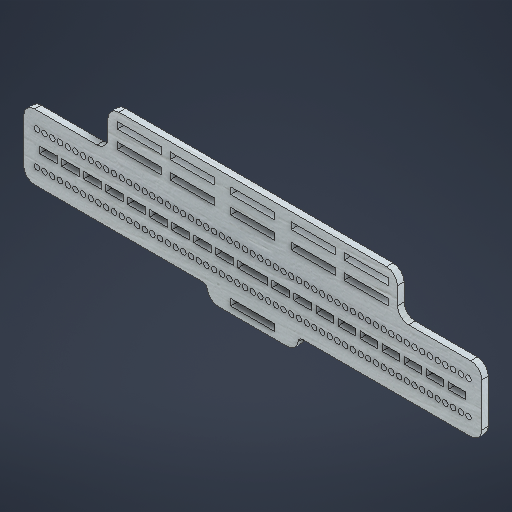
# Autodesk Inventor part: side_frame_test
Saved by Autodesk Inventor 2025.3 (Build 293356030, 356C)
## iProperties
Created: 2025-09-04
Part Number: side_frame_test
Material: 木材 (楓木)
Document SubType Name: Modeling
Designer: 陳泓任
Density: 0.67 g/cm^3
Appearance: 木材 - 白色刷漆
Author: 陳泓任
Autodesk Inventor part; units mm, degrees
ref_plane "YZ Plane" through (0, 0, 0) normal (1, 0, 0) x (0, 1, 0)
ref_plane "XZ Plane" through (0, 0, 0) normal (0, 1, 0) x (-1, 0, 0)
ref_plane "XY Plane" through (0, 0, 0) normal (0, 0, 1) x (1, 0, 0)
sketch "草圖1" plane through (0, 0, 0) normal (0, 0, 1) x (1, 0, 0)
  line L0 (41.49, 17.7685) -> (41.49, 20.7685)
  line L1 (41.49, 20.7685) -> (61.49, 20.7685)
  line L2 (61.49, 20.7685) -> (61.49, 17.7685)
  line L3 (61.49, 17.7685) -> (41.49, 17.7685)
  arc A0 (99, -14.8985) -> (104, -9.8985) centre (99, -9.8985) ccw
  arc A1 (-104, -9.8985) -> (-99, -14.8985) centre (-99, -9.8985) ccw
  line L4 (-61.49, 17.7685) -> (-61.49, 20.7685)
  line L5 (-61.49, 20.7685) -> (-41.49, 20.7685)
  line L6 (-41.49, 20.7685) -> (-41.49, 17.7685)
  line L7 (-41.49, 17.7685) -> (-61.49, 17.7685)
  arc A2 (65.74, 27.7685) -> (60.74, 32.7685) centre (60.74, 27.7685) ccw
  circle A3 centre (0, 7.5) radius 1.25
  circle A4 centre (0, -7.5) radius 1.25
  arc A5 (-70.74, 14.8985) -> (-65.74, 19.8985) centre (-70.74, 19.8985) ccw
  arc A6 (104, 9.8985) -> (99, 14.8985) centre (99, 9.8985) ccw
  arc A7 (-99, 14.8985) -> (-104, 9.8985) centre (-99, 9.8985) ccw
  arc A8 (65.74, 19.8985) -> (70.74, 14.8985) centre (70.74, 19.8985) ccw
  line L8 (-99, -14.8985) -> (-22.615, -14.8985)
  arc A9 (15.6624, -21.0852) -> (20.6286, -16.6661) centre (15.6624, -16.0852) ccw
  arc A10 (22.615, -14.8985) -> (20.6286, -16.6661) centre (22.615, -16.8985) ccw
  line L9 (-10, -18.0852) -> (-10, -15.0852)
  line L10 (-10, -15.0852) -> (10, -15.0852)
  line L11 (10, -15.0852) -> (10, -18.0852)
  line L12 (10, -18.0852) -> (-10, -18.0852)
  arc A11 (-20.6286, -16.6661) -> (-22.615, -14.8985) centre (-22.615, -16.8985) ccw
  arc A12 (-20.6286, -16.6661) -> (-15.6624, -21.0852) centre (-15.6624, -16.0852) ccw
  line L13 (-65.74, 27.7685) -> (-65.74, 19.8985)
  line L14 (-104, 9.8985) -> (-104, -9.8985)
  line L15 (104, 9.8985) -> (104, -9.8985)
  line L16 (-15.6624, -21.0852) -> (15.6624, -21.0852)
  line L17 (22.615, -14.8985) -> (99, -14.8985)
  line L18 (70.74, 14.8985) -> (99, 14.8985)
  line L19 (-99, 14.8985) -> (-70.74, 14.8985)
  line L20 (0, -35.3826) -> (0, 51.5191) construction
  line L21 (-104.9871, 0) -> (119.3176, 0) construction
  line L22 (65.74, 27.7685) -> (65.74, 19.8985)
  line L23 (0, 7.5) -> (0, -7.5)
  line L24 (-60.74, 32.7685) -> (60.74, 32.7685)
  arc A13 (-60.74, 32.7685) -> (-65.74, 27.7685) centre (-60.74, 27.7685) ccw
  line L25 (-61.49, 28.7685) -> (-41.49, 28.7685)
  line L26 (-61.49, 25.7685) -> (-61.49, 28.7685)
  line L27 (-41.49, 25.7685) -> (-61.49, 25.7685)
  line L28 (-41.49, 28.7685) -> (-41.49, 25.7685)
  line L29 (41.49, 28.7685) -> (61.49, 28.7685)
  line L30 (41.49, 25.7685) -> (41.49, 28.7685)
  line L31 (61.49, 25.7685) -> (41.49, 25.7685)
  line L32 (61.49, 28.7685) -> (61.49, 25.7685)
  line L33 (-17.49, 28.7685) -> (-17.49, 25.7685)
  line L34 (-17.49, 25.7685) -> (-37.49, 25.7685)
  line L35 (-37.49, 28.7685) -> (-17.49, 28.7685)
  line L36 (-37.49, 25.7685) -> (-37.49, 28.7685)
  line L37 (-17.49, 20.7685) -> (-17.49, 17.7685)
  line L38 (-17.49, 17.7685) -> (-37.49, 17.7685)
  line L39 (-37.49, 20.7685) -> (-17.49, 20.7685)
  line L40 (-37.49, 17.7685) -> (-37.49, 20.7685)
  line L41 (17.49, 28.7685) -> (17.49, 25.7685)
  line L42 (17.49, 25.7685) -> (37.49, 25.7685)
  line L43 (37.49, 28.7685) -> (17.49, 28.7685)
  line L44 (37.49, 25.7685) -> (37.49, 28.7685)
  line L45 (17.49, 20.7685) -> (17.49, 17.7685)
  line L46 (17.49, 17.7685) -> (37.49, 17.7685)
  line L47 (37.49, 20.7685) -> (17.49, 20.7685)
  line L48 (37.49, 17.7685) -> (37.49, 20.7685)
  line L49 (10, 28.7685) -> (10, 25.7685)
  line L50 (10, 25.7685) -> (-10, 25.7685)
  line L51 (-10, 28.7685) -> (10, 28.7685)
  line L52 (-10, 25.7685) -> (-10, 28.7685)
  line L53 (10, 20.7685) -> (10, 17.7685)
  line L54 (10, 17.7685) -> (-10, 17.7685)
  line L55 (-10, 20.7685) -> (10, 20.7685)
  line L56 (-10, 17.7685) -> (-10, 20.7685)
  circle A14 centre (3.5, 7.5) radius 1.25
  circle A15 centre (3.5, -7.5) radius 1.25
  circle A16 centre (-3.5, 7.5) radius 1.25
  circle A17 centre (-3.5, -7.5) radius 1.25
  circle A18 centre (7, 7.5) radius 1.25
  circle A19 centre (7, -7.5) radius 1.25
  circle A20 centre (-7, 7.5) radius 1.25
  circle A21 centre (-7, -7.5) radius 1.25
  circle A22 centre (10.5, 7.5) radius 1.25
  circle A23 centre (10.5, -7.5) radius 1.25
  circle A24 centre (-10.5, 7.5) radius 1.25
  circle A25 centre (-10.5, -7.5) radius 1.25
  circle A26 centre (14, 7.5) radius 1.25
  circle A27 centre (14, -7.5) radius 1.25
  circle A28 centre (-14, 7.5) radius 1.25
  circle A29 centre (-14, -7.5) radius 1.25
  circle A30 centre (17.5, 7.5) radius 1.25
  circle A31 centre (17.5, -7.5) radius 1.25
  circle A32 centre (-17.5, 7.5) radius 1.25
  circle A33 centre (-17.5, -7.5) radius 1.25
  circle A34 centre (21, 7.5) radius 1.25
  circle A35 centre (21, -7.5) radius 1.25
  circle A36 centre (-21, 7.5) radius 1.25
  circle A37 centre (-21, -7.5) radius 1.25
  circle A38 centre (24.5, 7.5) radius 1.25
  circle A39 centre (24.5, -7.5) radius 1.25
  circle A40 centre (-24.5, 7.5) radius 1.25
  circle A41 centre (-24.5, -7.5) radius 1.25
  circle A42 centre (28, 7.5) radius 1.25
  circle A43 centre (28, -7.5) radius 1.25
  circle A44 centre (-28, 7.5) radius 1.25
  circle A45 centre (-28, -7.5) radius 1.25
  circle A46 centre (31.5, 7.5) radius 1.25
  circle A47 centre (31.5, -7.5) radius 1.25
  circle A48 centre (-31.5, 7.5) radius 1.25
  circle A49 centre (-31.5, -7.5) radius 1.25
  circle A50 centre (35, 7.5) radius 1.25
  circle A51 centre (35, -7.5) radius 1.25
  circle A52 centre (-35, 7.5) radius 1.25
  circle A53 centre (-35, -7.5) radius 1.25
  circle A54 centre (38.5, 7.5) radius 1.25
  circle A55 centre (38.5, -7.5) radius 1.25
  circle A56 centre (-38.5, 7.5) radius 1.25
  circle A57 centre (-38.5, -7.5) radius 1.25
  circle A58 centre (42, 7.5) radius 1.25
  circle A59 centre (42, -7.5) radius 1.25
  circle A60 centre (-42, 7.5) radius 1.25
  circle A61 centre (-42, -7.5) radius 1.25
  circle A62 centre (45.5, 7.5) radius 1.25
  circle A63 centre (45.5, -7.5) radius 1.25
  circle A64 centre (-45.5, 7.5) radius 1.25
  circle A65 centre (-45.5, -7.5) radius 1.25
  circle A66 centre (49, 7.5) radius 1.25
  circle A67 centre (49, -7.5) radius 1.25
  circle A68 centre (-49, 7.5) radius 1.25
  circle A69 centre (-49, -7.5) radius 1.25
  circle A70 centre (52.5, 7.5) radius 1.25
  circle A71 centre (52.5, -7.5) radius 1.25
  circle A72 centre (-52.5, 7.5) radius 1.25
  circle A73 centre (-52.5, -7.5) radius 1.25
  circle A74 centre (56, 7.5) radius 1.25
  circle A75 centre (56, -7.5) radius 1.25
  circle A76 centre (-56, 7.5) radius 1.25
  circle A77 centre (-56, -7.5) radius 1.25
  circle A78 centre (59.5, 7.5) radius 1.25
  circle A79 centre (59.5, -7.5) radius 1.25
  circle A80 centre (-59.5, 7.5) radius 1.25
  circle A81 centre (-59.5, -7.5) radius 1.25
  circle A82 centre (63, 7.5) radius 1.25
  circle A83 centre (63, -7.5) radius 1.25
  circle A84 centre (-63, 7.5) radius 1.25
  circle A85 centre (-63, -7.5) radius 1.25
  circle A86 centre (66.5, 7.5) radius 1.25
  circle A87 centre (66.5, -7.5) radius 1.25
  circle A88 centre (-66.5, 7.5) radius 1.25
  circle A89 centre (-66.5, -7.5) radius 1.25
  circle A90 centre (70, 7.5) radius 1.25
  circle A91 centre (70, -7.5) radius 1.25
  circle A92 centre (-70, 7.5) radius 1.25
  circle A93 centre (-70, -7.5) radius 1.25
  circle A94 centre (73.5, 7.5) radius 1.25
  circle A95 centre (73.5, -7.5) radius 1.25
  circle A96 centre (-73.5, 7.5) radius 1.25
  circle A97 centre (-73.5, -7.5) radius 1.25
  circle A98 centre (77, 7.5) radius 1.25
  circle A99 centre (77, -7.5) radius 1.25
  circle A100 centre (-77, 7.5) radius 1.25
  circle A101 centre (-77, -7.5) radius 1.25
  circle A102 centre (80.5, 7.5) radius 1.25
  circle A103 centre (80.5, -7.5) radius 1.25
  circle A104 centre (-80.5, 7.5) radius 1.25
  circle A105 centre (-80.5, -7.5) radius 1.25
  circle A106 centre (84, 7.5) radius 1.25
  circle A107 centre (84, -7.5) radius 1.25
  circle A108 centre (-84, 7.5) radius 1.25
  circle A109 centre (-84, -7.5) radius 1.25
  circle A110 centre (87.5, 7.5) radius 1.25
  circle A111 centre (87.5, -7.5) radius 1.25
  circle A112 centre (-87.5, 7.5) radius 1.25
  circle A113 centre (-87.5, -7.5) radius 1.25
  circle A114 centre (91, 7.5) radius 1.25
  circle A115 centre (91, -7.5) radius 1.25
  circle A116 centre (-91, 7.5) radius 1.25
  circle A117 centre (-91, -7.5) radius 1.25
  circle A118 centre (94.5, 7.5) radius 1.25
  circle A119 centre (94.5, -7.5) radius 1.25
  circle A120 centre (-94.5, 7.5) radius 1.25
  circle A121 centre (-94.5, -7.5) radius 1.25
  circle A122 centre (98, 7.5) radius 1.25
  circle A123 centre (98, -7.5) radius 1.25
  circle A124 centre (-98, 7.5) radius 1.25
  circle A125 centre (-98, -7.5) radius 1.25
  point P0 (0, 0)
  point P1 (-65.74, 32.7685)
  point P2 (0, -15.0852)
  point P3 (-104, 0)
  point P4 (0, 32.7638)
  point P5 (-36.74, 27.7685)
  dimension "d0" = 20
  dimension "d1" = 3
  dimension "d2" = 3
  dimension "d4" = 2.5
  dimension "d7" = 4.25
  dimension "d11" = 5
  dimension "d12" = 2
  dimension "d16" = 15
  dimension "d26" = 29.797
  dimension "d29" = 45.23
  dimension "d30" = 31.3249
  dimension "d43" = 208
  dimension "d44" = 4.25
  dimension "d45" = 5
  dimension "d46" = 17.87
  dimension "d48" = 38.26
  dimension "d49" = 12
  dimension "d54" = 8
  dimension "d61" = 24
  dimension "d92" = 3.5
  constraints: 126 centre point, 114 end point, 24 point on circle, 22 tangent, 11 collinear, 10 equal length, 10 equal radius, 8 symmetric about line, 7 horizontal, 7 point on line, 5 perpendicular, 5 vertical, 2 midpoint, 262 other
  measures "d0" distance of L11.end L9.start
  measures "d1" distance of L9.start L9.end
  measures "d2" distance between parallel lines of L16 L12
  measures "d4" diameter of A3
  measures "d7" distance between parallel lines of L13 L4
  measures "d11" radius of A2
  measures "d12" radius of A11
  measures "d16" distance of L23.end L23.start
  measures "d26" distance between parallel lines of L18 L17
  measures "d29" distance of A10.centre A11.centre
  measures "d30" distance of L16.start L16.end
  measures "d43" diameter of L14 L20
  measures "d44" distance between parallel lines of L22 L2
  measures "d45" radius of A13
  measures "d46" distance between parallel lines of L19 L24
  measures "d48" distance between parallel lines of L22 L15
  measures "d49" distance between parallel lines of L5 L24
  measures "d54" distance of L4.end L25.start
  measures "d61" distance of L27.start L33.end
  measures "d92" distance of L23.start A14.centre
extrude "擠出1" add sketch "草圖1" along normal blind 3
sketch "草圖2" plane through (0, 0, 3) normal (0, 0, 1) x (1, 0, 0)
  line L0 (-104.9871, 0) -> (119.3176, 0) projected
  line L1 (0, -35.3826) -> (0, 51.5191) projected
  line L2 (-1.25, 1.5) -> (6.75, 1.5)
  line L3 (6.75, 1.5) -> (6.75, -1.5)
  line L4 (6.75, -1.5) -> (-1.25, -1.5)
  line L5 (-1.25, -1.5) -> (-1.25, 1.5)
  circle A0 centre (0, 7.5) radius 1.25 projected
  circle A1 centre (0, -7.5) radius 1.25 projected
  line L6 (8.75, 1.5) -> (16.75, 1.5)
  line L7 (16.75, -1.5) -> (8.75, -1.5)
  line L8 (8.75, -1.5) -> (8.75, 1.5)
  line L9 (16.75, 1.5) -> (16.75, -1.5)
  line L10 (18.75, 1.5) -> (26.75, 1.5)
  line L11 (26.75, -1.5) -> (18.75, -1.5)
  line L12 (18.75, -1.5) -> (18.75, 1.5)
  line L13 (26.75, 1.5) -> (26.75, -1.5)
  line L14 (28.75, 1.5) -> (36.75, 1.5)
  line L15 (36.75, -1.5) -> (28.75, -1.5)
  line L16 (28.75, -1.5) -> (28.75, 1.5)
  line L17 (36.75, 1.5) -> (36.75, -1.5)
  line L18 (38.75, 1.5) -> (46.75, 1.5)
  line L19 (46.75, -1.5) -> (38.75, -1.5)
  line L20 (38.75, -1.5) -> (38.75, 1.5)
  line L21 (46.75, 1.5) -> (46.75, -1.5)
  line L22 (48.75, 1.5) -> (56.75, 1.5)
  line L23 (56.75, -1.5) -> (48.75, -1.5)
  line L24 (48.75, -1.5) -> (48.75, 1.5)
  line L25 (56.75, 1.5) -> (56.75, -1.5)
  line L26 (58.75, 1.5) -> (66.75, 1.5)
  line L27 (66.75, -1.5) -> (58.75, -1.5)
  line L28 (58.75, -1.5) -> (58.75, 1.5)
  line L29 (66.75, 1.5) -> (66.75, -1.5)
  line L30 (68.75, 1.5) -> (76.75, 1.5)
  line L31 (76.75, -1.5) -> (68.75, -1.5)
  line L32 (68.75, -1.5) -> (68.75, 1.5)
  line L33 (76.75, 1.5) -> (76.75, -1.5)
  line L34 (1.25, 1.5) -> (-6.75, 1.5)
  line L35 (-6.75, 1.5) -> (-6.75, -1.5)
  line L36 (-6.75, -1.5) -> (1.25, -1.5)
  line L37 (1.25, -1.5) -> (1.25, 1.5)
  line L38 (-8.75, 1.5) -> (-16.75, 1.5)
  line L39 (-16.75, -1.5) -> (-8.75, -1.5)
  line L40 (-8.75, -1.5) -> (-8.75, 1.5)
  line L41 (-16.75, 1.5) -> (-16.75, -1.5)
  line L42 (-18.75, 1.5) -> (-26.75, 1.5)
  line L43 (-26.75, -1.5) -> (-18.75, -1.5)
  line L44 (-18.75, -1.5) -> (-18.75, 1.5)
  line L45 (-26.75, 1.5) -> (-26.75, -1.5)
  line L46 (-28.75, 1.5) -> (-36.75, 1.5)
  line L47 (-36.75, -1.5) -> (-28.75, -1.5)
  line L48 (-28.75, -1.5) -> (-28.75, 1.5)
  line L49 (-36.75, 1.5) -> (-36.75, -1.5)
  line L50 (-38.75, 1.5) -> (-46.75, 1.5)
  line L51 (-46.75, -1.5) -> (-38.75, -1.5)
  line L52 (-38.75, -1.5) -> (-38.75, 1.5)
  line L53 (-46.75, 1.5) -> (-46.75, -1.5)
  line L54 (-48.75, 1.5) -> (-56.75, 1.5)
  line L55 (-56.75, -1.5) -> (-48.75, -1.5)
  line L56 (-48.75, -1.5) -> (-48.75, 1.5)
  line L57 (-56.75, 1.5) -> (-56.75, -1.5)
  line L58 (-58.75, 1.5) -> (-66.75, 1.5)
  line L59 (-66.75, -1.5) -> (-58.75, -1.5)
  line L60 (-58.75, -1.5) -> (-58.75, 1.5)
  line L61 (-66.75, 1.5) -> (-66.75, -1.5)
  line L62 (-68.75, 1.5) -> (-76.75, 1.5)
  line L63 (-76.75, -1.5) -> (-68.75, -1.5)
  line L64 (-68.75, -1.5) -> (-68.75, 1.5)
  line L65 (-76.75, 1.5) -> (-76.75, -1.5)
  line L66 (78.75, 1.5) -> (86.75, 1.5)
  line L67 (86.75, -1.5) -> (78.75, -1.5)
  line L68 (78.75, -1.5) -> (78.75, 1.5)
  line L69 (86.75, 1.5) -> (86.75, -1.5)
  line L70 (88.75, 1.5) -> (96.75, 1.5)
  line L71 (96.75, -1.5) -> (88.75, -1.5)
  line L72 (88.75, -1.5) -> (88.75, 1.5)
  line L73 (96.75, 1.5) -> (96.75, -1.5)
  line L74 (-78.75, 1.5) -> (-86.75, 1.5)
  line L75 (-86.75, -1.5) -> (-78.75, -1.5)
  line L76 (-78.75, -1.5) -> (-78.75, 1.5)
  line L77 (-86.75, 1.5) -> (-86.75, -1.5)
  line L78 (-88.75, 1.5) -> (-96.75, 1.5)
  line L79 (-96.75, -1.5) -> (-88.75, -1.5)
  line L80 (-88.75, -1.5) -> (-88.75, 1.5)
  line L81 (-96.75, 1.5) -> (-96.75, -1.5)
  point P0 (0, 0)
  point P1 (-1.25, 0)
  point P2 (8.75, 0)
  point P3 (18.75, 0)
  point P4 (28.75, 0)
  point P5 (38.75, 0)
  point P6 (48.75, 0)
  point P7 (58.75, 0)
  point P8 (68.75, 0)
  point P9 (1.25, 0)
  point P10 (-8.75, 0)
  point P11 (-18.75, 0)
  point P12 (-28.75, 0)
  point P13 (-38.75, 0)
  point P14 (-48.75, 0)
  point P15 (-58.75, 0)
  point P16 (-68.75, 0)
  point P17 (-68.75, 0)
  point P18 (-76.75, 0)
  point P19 (78.75, 0)
  point P20 (88.75, 0)
  dimension "d33" = 3
  dimension "d34" = 8
  dimension "d38" = 10
  constraints: 160 end point, 48 symmetric about line, 2 horizontal, 2 parallel, 1 midpoint, 1 perpendicular, 1 tangent, 82 other
  measures "d33" distance of L2.end L3.end
  measures "d34" distance of L3.end L4.end
  measures "d38" distance of L2.start L6.start
extrude "擠出2" cut sketch "草圖2" against normal up to surface (3 mm away) contours L81 L78 L80 L0 | L0 L80 L79 L81 | L77 L74 L76 L0 | L0 L76 L75 L77 | L65 L62 L64 L0 | L0 L64 L63 L65 | L61 L58 L60 L0 | L0 L60 L59 L61 | L57 L54 L56 L0 | L0 L56 L55 L57 | L53 L50 L52 L0 | L0 L52 L51 L53 | L49 L46 L48 L0 | L0 L48 L47 L49 | L45 L42 L44 L0 | L0 L44 L43 L45 | L41 L38 L40 L0 | L0 L40 L39 L41 | L35 L34 L5 L0 | L0 L5 L36 L35 | L5 L2 L1 L0 | L0 L1 L4 L5 | L1 L2 L37 L0 | L0 L37 L4 L1 | L37 L2 L3 L0 | L0 L3 L4 L37 | L8 L6 L9 L0 | L0 L9 L7 L8 | L12 L10 L13 L0 | L0 L13 L11 L12 | L16 L14 L17 L0 | L0 L17 L15 L16 | L20 L18 L21 L0 | L0 L21 L19 L20 | L24 L22 L25 L0 | L0 L25 L23 L24 | L28 L26 L29 L0 | L0 L29 L27 L28 | L32 L30 L33 L0 | L0 L33 L31 L32 | L68 L66 L69 L0 | L0 L69 L67 L68 | L72 L70 L73 L0 | L0 L73 L71 L72
sketch "草圖3" plane through (0, 0, 3) normal (0, 0, 1) x (1, 0, 0)
  line L0 (0, 52.3829) -> (0, -39.0235)
  line L1 (-112.5881, 0) -> (123.4866, 0)
  point P0 (0, 0)
  constraints: 4 end point, 2 point on line, 1 horizontal, 1 vertical
